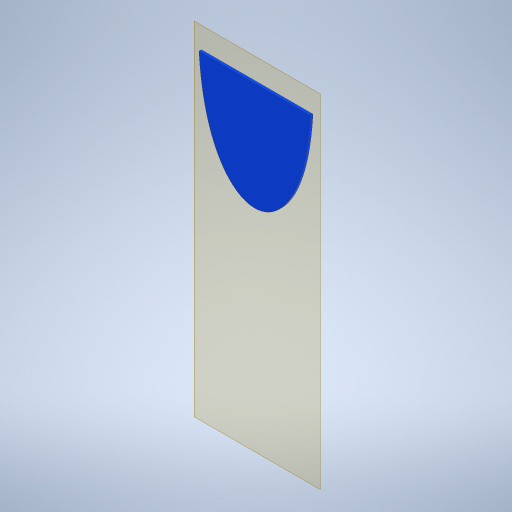
# Autodesk Inventor part: back-flaps
Saved by Autodesk Inventor 2023 (Build 270158030, 158C)
## iProperties
Created: 2024-09-10
Part Number: back-flaps
Material: Generic
Document SubType Name: Modeling
Designer: Imogen Heard
Density: 1 g/cm^3
Appearance: Default
Author: Imogen Heard
Autodesk Inventor part; units mm, degrees
ref_plane "YZ Plane" through (0, 0, 0) normal (1, 0, 0) x (0, 1, 0)
ref_plane "XZ Plane" through (0, 0, 0) normal (0, 1, 0) x (-1, 0, 0)
ref_plane "XY Plane" through (0, 0, 0) normal (0, 0, 1) x (1, 0, 0)
ref_plane "Work Plane1" through (0, 0, 0) normal (0, 0, 1) x (1, 0, 0)
sketch "Sketch1" plane through (0, 0, 0) normal (0, 0, 1) x (1, 0, 0)
  line L0 (0, 0) -> (700, 0) projected
  line L1 (700, 0) -> (700, 1930) projected
  line L2 (0, 1930) -> (700, 1930) projected
  line L3 (0, 0) -> (0, 1930) projected
  line L4 (700, 1920) -> (660, 1230) construction
  line L5 (40, 1230) -> (0, 1920) construction
  spline S0 degree 4 poles (700, 1920) (660, 1230) (350, 1030) (40, 1230) (0, 1920) knots 1 1 1 1 1 2 2 2 2 2
  line L6 (660, 1230) -> (350, 1030) construction
  line L7 (350, 1030) -> (40, 1230) construction
  line L8 (699.3756, 1930) -> (0, 1930)
  line L9 (0, 1930) -> (0, 1920)
  line L10 (0, 1920) -> (700, 1920)
  line L11 (700, 1920) -> (700, 1930)
  point P0 (0, 1920)
  dimension "d0" = 700
  dimension "d1" = 900
  dimension "d2" = 350
  dimension "d3" = 350
  dimension "d4" = 40
  dimension "d5" = 40
  dimension "d8" = 10
  constraints: 8 end point, 2 coincident, 2 parallel, 1 horizontal, 1 horizontal alignment, 1 perpendicular, 1 point on line, 3 other
  measures "d0" distance from line of L4.end L2
  measures "d1" distance from line of L2 L6.end
  measures "d2" distance from line of L3 L6.end
  measures "d3" distance from line of L1 L6.end
  measures "d4" distance from line of L3 L5.start
  measures "d5" distance from line of L1 L4.end
  measures "d8" distance between parallel lines of L2 L10
extrude "Extrusion1" add sketch "Sketch1" along normal blind 15 contours L10 S0
body "Solid1"
